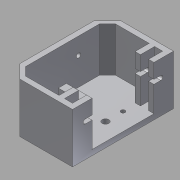
# Autodesk Inventor part: case-new
Saved by Autodesk Inventor 2014 (Build 180170000, 170)
## iProperties
Created: 2014-10-07
Part Number: case-new
Material: 一般
Document SubType Name: Modeling
Designer: kayako
Density: 1 g/cm^3
Appearance: 滑らか - 白
Author: kayako
Autodesk Inventor part; units mm, degrees
ref_plane "YZ Plane" through (0, 0, 0) normal (1, 0, 0) x (0, 1, 0)
ref_plane "XZ Plane" through (0, 0, 0) normal (0, 1, 0) x (-1, 0, 0)
ref_plane "XY Plane" through (0, 0, 0) normal (0, 0, 1) x (1, 0, 0)
sketch "スケッチ1" plane through (0, 0, 0) normal (0, 0, 1) x (1, 0, 0)
  line L0 (-26.25, 0) -> (26.25, 0) construction
  line L1 (0, -17.15) -> (0, 17.15) construction
  line L2 (-18.75, 12.25) -> (18.75, 12.25)
  line L3 (18.75, 12.25) -> (18.75, -7.25)
  line L4 (13.75, -12.25) -> (-13.75, -12.25)
  line L5 (-18.75, -7.25) -> (-18.75, 12.25)
  line L6 (-13.75, -12.25) -> (-18.75, -7.25)
  line L7 (18.75, -7.25) -> (13.75, -12.25)
  point P0 (0, 0)
  point P1 (18.75, -12.25)
  point P2 (-18.75, -12.25)
  dimension "d0" = 37.5
  dimension "d1" = 24.5
  dimension "d2" = 18.75
  dimension "d3" = 12.25
  dimension "d76" = 5
  dimension "d77" = 5
  dimension "d78" = 5
  dimension "d79" = 5
  constraints: 12 end point, 4 point on line, 2 parallel, 1 horizontal, 1 perpendicular
  measures "d0" distance of L2.start L2.end
  measures "d1" distance of L2.end point (18.75, -12.25)
  measures "d2" distance between parallel lines of L3 L1
  measures "d3" distance between parallel lines of L0 L4
  measures "d76" distance of L4.end point (-18.75, -12.25)
  measures "d77" distance of L5.start point (-18.75, -12.25)
  measures "d78" distance of L3.end point (18.75, -12.25)
  measures "d79" distance of L4.start point (18.75, -12.25)
extrude "押し出し1" add sketch "スケッチ1" along normal blind 18.5
sketch "スケッチ2" plane through (0, 0, 18.5) normal (0, 0, 1) x (1, 0, 0)
  line L0 (18.75, 12.25) -> (-18.75, 12.25) projected
  line L1 (-18.75, 12.25) -> (-18.75, -7.25) projected
  line L2 (-13.75, -12.25) -> (13.75, -12.25) projected
  line L3 (18.75, -7.25) -> (18.75, 12.25) projected
  line L4 (16.75, 10.25) -> (16.75, -7.25)
  line L5 (13.75, -10.25) -> (-13.75, -10.25)
  line L6 (-16.75, -7.25) -> (-16.75, 10.25)
  line L7 (-11.5, 12.25) -> (11.5, 12.25)
  line L8 (11.5, 12.25) -> (11.5, 10.25)
  line L9 (-11.5, 10.25) -> (-11.5, 12.25)
  line L10 (-16.75, 10.25) -> (-11.5, 10.25)
  line L11 (11.5, 10.25) -> (16.75, 10.25)
  line L12 (-16.75, -7.25) -> (-13.75, -10.25)
  line L13 (16.75, -7.25) -> (13.75, -10.25)
  point P0 (-18.75, -12.25)
  point P1 (18.75, -12.25)
  point P2 (0, 0)
  dimension "d6" = 2
  dimension "d7" = 7.25
  dimension "d8" = 7.25
  dimension "d66" = 5
  dimension "d67" = 5
  dimension "d68" = 5
  dimension "d69" = 5
  dimension "d71" = 2
  dimension "d72" = 2
  dimension "d74" = 2
  dimension "d75" = 2
  constraints: 20 end point, 2 horizontal, 2 perpendicular, 1 parallel, 1 point on line
  measures "d6" distance between parallel lines of L1 L6
  measures "d7" distance between parallel lines of L9 L1
  measures "d8" distance between parallel lines of L3 L8
  measures "d66" distance from line of L2 L6.start
  measures "d67" distance from line of L1 L5.end
  measures "d68" distance from line of L3 L5.start
  measures "d69" distance from line of L4.end L2
  measures "d71" distance between parallel lines of L2 L5
  measures "d72" distance from line of L3 L4.start
  measures "d74" distance between parallel lines of L11 L0
  measures "d75" distance between parallel lines of L10 L0
extrude "押し出し2" cut sketch "スケッチ2" against normal blind 16.5
sketch "スケッチ3" plane through (0, 0, 2) normal (0, 0, 1) x (1, 0, 0)
  line L0 (13.75, -10.25) -> (-13.75, -10.25) projected
  line L1 (-1.5, -10.25) -> (1.5, -10.25)
  line L2 (1.5, -10.25) -> (1.5, -1.75)
  line L3 (1.5, -1.75) -> (-1.5, -1.75)
  line L4 (-1.5, -1.75) -> (-1.5, -10.25)
  point P0 (0, 0)
  dimension "d11" = 3
  dimension "d12" = 8.5
  dimension "d13" = 1.5
  constraints: 8 end point, 2 parallel, 1 horizontal, 1 perpendicular, 1 point on line
  measures "d11" distance of L3.end L2.end
  measures "d12" distance of L2.end L1.end
  measures "d13" distance from line of L4 point (0, 0)
extrude "押し出し3" add sketch "スケッチ3" along normal blind 3.5
sketch "スケッチ4" plane through (-16.75, 10.25, 18.5) normal (0, -1, 0) x (1, 0, 0)
  line L0 (0, 0) -> (5.25, 0) projected
  line L1 (5.25, 0) -> (5.25, -16.5) projected
  point P0 (16.75, -18.5)
  point P1 (2.75, -6.25)
  dimension "d16" = 6.25
  dimension "d50" = 2.5
  measures "d16" distance from line of point (2.75, -6.25) L0
  measures "d50" distance from line of L1 point (2.75, -6.25)
hole "穴1" at (-14, 10.25, 12.25) direction (0, 1, 0) diameter 1.6 end through all
mirror "ミラー1" about plane through (0, 0, 0) normal (1, 0, 0) of "穴1"
sketch "スケッチ5" plane through (-18.75, -12.25, 0) normal (0, -1, 0) x (1, 0, 0)
  circle A0 centre (4.75, 12.25) radius 0.8 projected
  line L0 (5, 18.5) -> (32.5, 18.5) projected
  point P0 (18.75, 0)
  point P1 (12.75, 12.25)
  point P2 (37.5, 18.5)
  point P3 (0, 18.5)
  dimension "d25" = 8
  dimension "d60" = 6.25
  measures "d25" distance of A0.centre point (12.75, 12.25)
  measures "d60" distance from line of L0 A0.centre
hole "穴2" at (-6, -12.25, 12.25) direction (0, 1, 0) diameter 1.6 end through all
sketch "スケッチ6" plane through (0, 0, 2) normal (0, 0, 1) x (1, 0, 0)
  line L0 (-1.5, -10.25) -> (-13.75, -10.25) projected
  point P0 (0, 0)
  point P1 (0, 5.75)
  dimension "d33" = 16
  measures "d33" distance from line of point (0, 5.75) L0
hole "穴3" at (0, 5.75, 2) direction (0, 0, -1) diameter 2.5 end through all
sketch "スケッチ7" plane through (0, 0, 2) normal (0, 0, 1) x (1, 0, 0)
  circle A0 centre (0, 5.75) radius 1.25 projected
  point P0 (0, 0)
  point P1 (-6.5, 5.75)
  point P2 (-12.5, 5.75)
  dimension "d41" = 6.5
  dimension "d42" = 12.5
  constraints: 2 horizontal alignment
  measures "d41" distance of A0.centre point (-6.5, 5.75)
  measures "d42" distance of A0.centre point (-12.5, 5.75)
hole "穴4" at (-6.5, 5.75, 2) at (-12.5, 5.75, 2) direction (0, 0, -1) diameter 1.6 end through all
mirror "ミラー2" about plane through (0, 0, 0) normal (1, 0, 0) of "穴4"
sketch "スケッチ8" plane through (0, 0, 2) normal (0, 0, 1) x (1, 0, 0)
  line L0 (-16.75, 10.25) -> (-11.5, 10.25) projected
  line L1 (-16.75, -10.25) -> (-16.75, 10.25) projected
  line L2 (-16.75, 7.25) -> (-11.5, 7.25)
  line L3 (-11.5, 7.25) -> (-11.5, 5.25)
  line L4 (-11.5, 5.25) -> (-16.75, 5.25)
  line L5 (-16.75, 5.25) -> (-16.75, 7.25)
  point P0 (-13.75, -10.25)
  point P1 (0, 0)
  dimension "d51" = 2
  dimension "d52" = 5.25
  dimension "d53" = 3
  constraints: 8 end point, 2 parallel, 1 horizontal, 1 perpendicular, 2 other
  measures "d51" distance of L2.end L3.end
  measures "d52" distance of L2.start L2.end
  measures "d53" distance between parallel lines of L2 L0
extrude "押し出し4" add sketch "スケッチ8" along normal blind 16.5
sketch "スケッチ9" plane through (-16.75, 5.25, 2) normal (0, -1, 0) x (1, 0, 0)
  circle A0 centre (2.75, 10.25) radius 0.8 projected
  point P0 (16.75, -2)
extrude "押し出し5" cut sketch "スケッチ9" against normal blind 3
mirror "ミラー3" about plane through (0, 0, 0) normal (1, 0, 0) of "押し出し4"
mirror "ミラー4" about plane through (0, 0, 0) normal (1, 0, 0) of "押し出し5"
sketch "スケッチ10" plane through (-18.75, 12.25, 0) normal (0, 1, 0) x (1, 0, 0)
  circle A0 centre (4.75, -12.25) radius 0.8 projected
  line L0 (7.25, -18.5) -> (7.25, -2) projected
  line L1 (4.75, -11.45) -> (7.25, -11.45)
  line L2 (7.25, -11.45) -> (7.25, -13.05)
  line L3 (7.25, -13.05) -> (4.75, -13.05)
  line L4 (4.75, -13.05) -> (4.75, -11.45)
  point P0 (18.75, 0)
  constraints: 8 end point, 2 horizontal, 2 parallel, 1 perpendicular, 1 point on line, 1 vertical alignment, 1 other
extrude "押し出し6" cut sketch "スケッチ10" against normal blind 10 contours A0 L4 | A0 L1 L0 L3 picked at (4.8657, -12.0097)
mirror "ミラー5" about plane through (0, 0, 0) normal (1, 0, 0) of "押し出し6"
equation "\"d2\" = 0.5 * d0"
equation "\"d3\" = 0.5 * d1"
equation "\"d77\" = d76"
equation "\"d78\" = d76"
equation "\"d79\" = d78"
equation "\"d8\" = d7"
equation "\"d13\" = 0.5 * d11"
